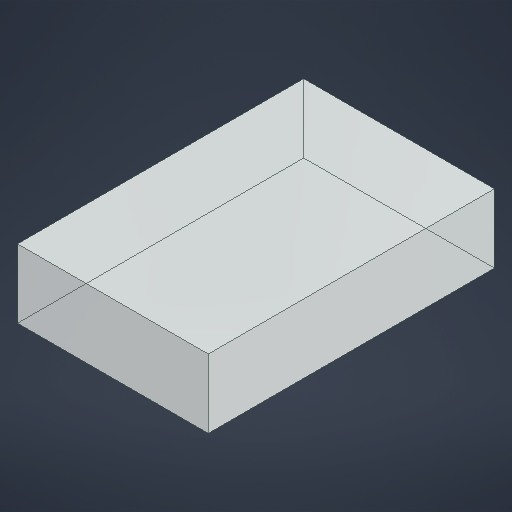
# Autodesk Inventor part: pcb_aproximace
Saved by Autodesk Inventor 2026 (Build 300175050, 175E)
## iProperties
Created: 2026-03-25
Part Number: pcb_aproximace
Material: Glass
Document SubType Name: Modeling
Designer: josef
Mass: 122.625 g
Surface Area: 112.5 cm^2
Volume: 56.25 cm^3
Density: 2.18 g/cm^3
Appearance: Clear
Author: josef
Autodesk Inventor part; units mm, degrees
ref_plane "YZ Plane" through (0, 0, 0) normal (1, 0, 0) x (0, 1, 0)
ref_plane "XZ Plane" through (0, 0, 0) normal (0, 1, 0) x (-1, 0, 0)
ref_plane "XY Plane" through (0, 0, 0) normal (0, 0, 1) x (1, 0, 0)
sketch "Sketch1" plane through (0, 0, 0) normal (0, 1, 0) x (-1, 0, 0)
  line L0 (28.2675, 14.5897) -> (-21.7325, 14.5897)
  line L1 (-21.7325, 14.5897) -> (-21.7325, -60.4103)
  line L2 (-21.7325, -60.4103) -> (28.2675, -60.4103)
  line L3 (28.2675, -60.4103) -> (28.2675, 14.5897)
  point P0 (0, 0)
  dimension "d0" = 75
  dimension "d1" = 50
  constraints: 8 end point, 2 parallel, 1 horizontal, 1 perpendicular
  measures "d0" distance of L2.end L0.start
  measures "d1" distance between parallel lines of L1 L3
extrude "Extrusion1" add sketch "Sketch1" along normal blind 18
body "Solid1"
